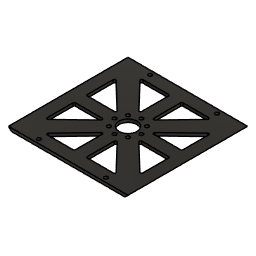
wall (Autodesk Fusion 360 design; units mm, degrees)
Autodesk Fusion 360 part; units mm, degrees
sketch "Sketch1" plane through (0, 0, 0) normal (0, 0, 1) x (1, 0, 0)
  line L0 (40, -40) -> (-60, -40)
  line L1 (-60, -40) -> (-60, 60)
  line L2 (-60, 60) -> (40, 60)
  line L3 (40, 60) -> (40, -40)
  dimension "d1" = 100
  dimension "d2" = 100
  constraint horizontal L0
  constraint vertical L1
  constraint horizontal L2
  constraint vertical L3
  measures "d1" distance of L0.start L0.end
  measures "d2" distance of L0.start L2.end
extrude "Extrude1" add sketch "Sketch1" along normal blind 2.5
sketch "Sketch2" plane through (0, 0, 2.5) normal (0, 0, 1) x (-1, 0, 0)
  line L0 (-40, -60) -> (60, -60)
  line L1 (60, -60) -> (60, 40)
  line L2 (60, 40) -> (-40, 40)
  line L3 (-40, 40) -> (-40, -60)
  point P0 (44.5, -10)
  point P1 (38, 36.5)
  point P2 (10, 36.5)
  point P3 (-18, 36.5)
  point P4 (-24.5, -10)
  point P5 (38, -56.5)
  point P6 (10, -56.5)
  point P7 (-18, -56.5)
  dimension "d7" = 50
  dimension "d11" = 50
  dimension "d12" = 28
  dimension "d13" = 28
  dimension "d14" = 3.5
  dimension "d15" = 3.5
  dimension "d16" = 3.5
  dimension "d17" = 50
  dimension "d25" = 50
  dimension "d26" = 28
  dimension "d27" = 28
  dimension "d28" = 3.5
  dimension "d29" = 3.5
  dimension "d30" = 3.5
  dimension "d34" = 15.5
  dimension "d35" = 15.5
  measures "d7" distance of L0 P0
  measures "d11" distance of L1 P2
  measures "d12" distance of P1 P2
  measures "d13" distance of P2 P3
  measures "d14" distance of L2 P1
  measures "d15" distance of L2 P2
  measures "d16" distance of L2 P3
  measures "d17" distance of L2 P4
  measures "d25" distance of L1 P6
  measures "d26" horizontal distance of P5 P6
  measures "d27" horizontal distance of P6 P7
  measures "d28" distance of L0 P6
  measures "d29" distance of L0 P5
  measures "d30" distance of L0 P7
  measures "d34" distance of L1 P0
  measures "d35" distance of L3 P4
hole "Hole1" at (-38, 56.5, 2.5) at (18, 56.5, 2.5) at (18, -36.5, 2.5) at (-38, -36.5, 2.5) direction (0, 0, -1) diameter 3 depth 10 tip angle 118
sketch "Sketch3" plane through (0, 0, 2.5) normal (0, 0, 1) x (-1, 0, 0)
  circle A0 centre (-18, 36.5) radius 1.5
  circle A1 centre (38, -56.5) radius 1.5
  circle A2 centre (-18, -56.5) radius 1.5
  circle A3 centre (38, 36.5) radius 1.5
  line L0 (-40, -60) -> (60, -60)
  line L1 (60, -60) -> (60, 40)
  line L2 (60, 40) -> (-40, 40)
  line L3 (-40, 40) -> (-40, -60)
  circle A4 centre (10, -10) radius 7.5
  dimension "d36" = 15
  measures "d36" diameter of A4
extrude "Extrude2" cut sketch "Sketch3" against normal blind 2.5 contours A4
sketch "Sketch4" plane through (0, 0, 0) normal (0, 0, 1) x (1, 0, 0)
  circle A0 centre (-10, 10) radius 15
  circle A1 centre (-10, 10) radius 7.5
  circle A2 centre (-10, 21.25) radius 1.5
  circle A3 centre (-2.045, 17.955) radius 1.5
  circle A4 centre (1.25, 10) radius 1.5
  circle A5 centre (-2.045, 2.045) radius 1.5
  circle A6 centre (-10, -1.25) radius 1.5
  circle A7 centre (-17.955, 2.045) radius 1.5
  circle A8 centre (-21.25, 10) radius 1.5
  circle A9 centre (-17.955, 17.955) radius 1.5
  point P0 (-10, 21.25)
  point P1 (-17.955, 17.955)
  point P2 (-21.25, 10)
  point P3 (-17.955, 2.045)
  point P4 (-10, -1.25)
  point P5 (-2.045, 2.045)
  point P6 (1.25, 10)
  point P7 (-2.045, 17.955)
  point P8 (-17.955, 17.955)
  point P9 (-21.25, 10)
  point P10 (-17.955, 2.045)
  point P11 (-10, -1.25)
  point P12 (-2.045, 2.045)
  point P13 (1.25, 10)
  point P14 (-2.045, 17.955)
  dimension "d39" = 30
  dimension "d40" = 11.25
  dimension "d42" = 360
  dimension "d46" = 3
  dimension "d47" = 3
  dimension "d48" = 3
  dimension "d49" = 3
  dimension "d50" = 3
  dimension "d51" = 3
  dimension "d52" = 3
  dimension "d53" = 3
  constraint coincident P0 A2.centre
  constraint coincident P14 P7
  constraint coincident P13 P6
  constraint coincident P12 P5
  constraint coincident P11 P4
  constraint coincident P10 P3
  constraint coincident P9 P2
  constraint coincident P8 P1
  measures "d39" diameter of A0
  measures "d40" distance of P0 A0.centre
  measures "d46" diameter of A2
  measures "d47" diameter of A3
  measures "d48" diameter of A4
  measures "d49" diameter of A5
  measures "d50" diameter of A6
  measures "d51" diameter of A7
  measures "d52" diameter of A8
  measures "d53" diameter of A9
extrude "Extrude3" cut sketch "Sketch4" along normal blind 9 contours A2 | A3 | A4 | A5 | A6 | A7 | A8 | A9
sketch "Sketch7" plane through (0, 0, 2.5) normal (0, 0, 1) x (-1, 0, 0)
  circle A0 centre (10, -21.25) radius 1.5
  circle A1 centre (10, 1.25) radius 1.5
  circle A2 centre (2.045, -2.045) radius 1.5
  circle A3 centre (17.955, -17.955) radius 1.5
  circle A4 centre (2.045, -17.955) radius 1.5
  circle A5 centre (17.955, -2.045) radius 1.5
  circle A6 centre (-1.25, -10) radius 1.5
  circle A7 centre (21.25, -10) radius 1.5
  circle A8 centre (10, -10) radius 7.5
  circle A9 centre (-18, 36.5) radius 1.5
  circle A10 centre (38, -56.5) radius 1.5
  circle A11 centre (-18, -56.5) radius 1.5
  circle A12 centre (38, 36.5) radius 1.5
  line L0 (-40, -60) -> (60, -60)
  line L1 (60, -60) -> (60, 40)
  line L2 (60, 40) -> (-40, 40)
  line L3 (-40, 40) -> (-40, -60)
  circle A13 centre (10, -10) radius 15
  dimension "d56" = 30
  constraint concentric A8 A13
  measures "d56" diameter of A13
sketch "Sketch8" plane through (0, 0, 2.5) normal (0, 0, 1) x (-1, 0, 0)
  line L0 (10, -10) -> (10, 40)
  line L1 (10, 40) -> (10, -60)
  constraint vertical L0
  constraint parallel L0 L1
sketch "Sketch9" plane through (0, 0, 2.5) normal (0, 0, 1) x (-1, 0, 0)
  line L0 (-40, -10) -> (60, -10)
  constraint horizontal L0
sketch "Sketch10" plane through (0, 0, 2.5) normal (0, 0, 1) x (-1, 0, 0)
  line L0 (-40, 40) -> (60, -60)
sketch "Sketch11" plane through (0, 0, 0) normal (0, 0, 1) x (1, 0, 0)
  line L0 (-60, -40) -> (40, 60)
sketch "Sketch13" plane through (0, 0, 2.5) normal (0, 0, 1) x (-1, 0, 0)
  line L0 (-17.6512, 30) -> (4, 30)
  line L1 (5, 29) -> (5, 6.4828)
  line L2 (3.2792, 5.7897) -> (-18.372, 28.3069)
  arc A0 (-17.6512, 30) -> (-18.372, 28.3069) centre (-17.6512, 29) ccw
  arc A1 (5, 29) -> (4, 30) centre (4, 29) ccw
  arc A2 (3.2792, 5.7897) -> (5, 6.4828) centre (4, 6.4828) ccw
  line L3 (-40, 40) -> (60, -60)
  arc A3 (-6.4828, -5) -> (-5.7897, -3.2792) centre (-6.4828, -4) ccw
  line L4 (-29, -5) -> (-6.4828, -5)
  line L5 (-5.7897, -3.2792) -> (-28.3069, 18.372)
  arc A4 (-28.3069, 18.372) -> (-30, 17.6512) centre (-29, 17.6512) ccw
  line L6 (-30, 17.6512) -> (-30, -4)
  arc A5 (-30, -4) -> (-29, -5) centre (-29, -4) ccw
  line L7 (-40, -10) -> (60, -10)
  line L8 (-29, -15) -> (-6.4828, -15)
  arc A6 (-5.7897, -16.7208) -> (-6.4828, -15) centre (-6.4828, -16) ccw
  line L9 (-5.7897, -16.7208) -> (-28.3069, -38.372)
  arc A7 (-30, -37.6512) -> (-28.3069, -38.372) centre (-29, -37.6512) ccw
  line L10 (-30, -37.6512) -> (-30, -16)
  arc A8 (-29, -15) -> (-30, -16) centre (-29, -16) ccw
  line L11 (60, 40) -> (-40, -60)
  line L12 (5, -49) -> (5, -26.4828)
  arc A9 (4, -50) -> (5, -49) centre (4, -49) ccw
  arc A10 (5, -26.4828) -> (3.2792, -25.7897) centre (4, -26.4828) ccw
  line L13 (3.2792, -25.7897) -> (-18.372, -48.3069)
  line L14 (-17.6512, -50) -> (4, -50)
  arc A11 (-18.372, -48.3069) -> (-17.6512, -50) centre (-17.6512, -49) ccw
  line L15 (10, 40) -> (10, -60)
  arc A12 (16.7208, -25.7897) -> (15, -26.4828) centre (16, -26.4828) ccw
  line L16 (15, -49) -> (15, -26.4828)
  line L17 (16.7208, -25.7897) -> (38.372, -48.3069)
  line L18 (37.6512, -50) -> (16, -50)
  arc A13 (15, -49) -> (16, -50) centre (16, -49) ccw
  arc A14 (37.6512, -50) -> (38.372, -48.3069) centre (37.6512, -49) ccw
  arc A15 (26.4828, -15) -> (25.7897, -16.7208) centre (26.4828, -16) ccw
  line L19 (25.7897, -16.7208) -> (48.3069, -38.372)
  line L20 (49, -15) -> (26.4828, -15)
  arc A16 (50, -16) -> (49, -15) centre (49, -16) ccw
  line L21 (50, -37.6512) -> (50, -16)
  arc A17 (48.3069, -38.372) -> (50, -37.6512) centre (49, -37.6512) ccw
  line L22 (25.7897, -3.2792) -> (48.3069, 18.372)
  arc A18 (50, 17.6512) -> (48.3069, 18.372) centre (49, 17.6512) ccw
  line L23 (50, 17.6512) -> (50, -4)
  arc A19 (49, -5) -> (50, -4) centre (49, -4) ccw
  line L24 (49, -5) -> (26.4828, -5)
  arc A20 (25.7897, -3.2792) -> (26.4828, -5) centre (26.4828, -4) ccw
  line L25 (37.6512, 30) -> (16, 30)
  arc A21 (38.372, 28.3069) -> (37.6512, 30) centre (37.6512, 29) ccw
  line L26 (16.7208, 5.7897) -> (38.372, 28.3069)
  arc A22 (15, 6.4828) -> (16.7208, 5.7897) centre (16, 6.4828) ccw
  line L27 (15, 29) -> (15, 6.4828)
  arc A23 (16, 30) -> (15, 29) centre (16, 29) ccw
  point P0 (-20, 30)
  point P1 (5, 30)
  point P2 (5, 4)
  dimension "d57" = 1
  constraint horizontal L0
  constraint perpendicular L0 L1
  constraint tangent L0 A0
  constraint tangent L2 A0
  constraint tangent L0 A1
  constraint tangent L1 A1
  constraint equal A0 A1
  constraint tangent L1 A2
  constraint tangent L2 A2
  constraint equal A0 A2
  constraint symmetric L0.start L3 A4.end
  constraint symmetric L2.end L3 L5.end
  constraint symmetric A0 L3 A4
  constraint symmetric L0.end L3 L6.end
  constraint symmetric L1.start L3 L4.start
  constraint symmetric A1 L3 A5
  constraint symmetric L1.end L3 A3.start
  constraint symmetric L2.start L3 A3.end
  constraint symmetric A2 L3 A3
  constraint symmetric A3.end L7 A6.start
  constraint symmetric A3.start L7 L8.end
  constraint symmetric A3 L7 A6
  constraint symmetric L4.start L7 L8.start
  constraint symmetric L5.end L7 L9.end
  constraint symmetric A4.end L7 A7.start
  constraint symmetric A4 L7 A7
  constraint symmetric L6.end L7 L10.end
  constraint symmetric A5 L7 A8
  constraint symmetric L8.start L11 L12.start
  constraint symmetric L8.end L11 L12.end
  constraint symmetric A6.start L11 A10.end
  constraint symmetric A6 L11 A10
  constraint symmetric L9.end L11 L13.end
  constraint symmetric A7.start L11 L14.start
  constraint symmetric A7 L11 A11
  constraint symmetric L10.end L11 A9.start
  constraint symmetric A8 L11 A9
  constraint symmetric L12.start L15 L16.start
  constraint symmetric L12.end L15 A12.end
  constraint symmetric A9.start L15 L18.end
  constraint symmetric A9 L15 A13
  constraint symmetric A10.end L15 A12.start
  constraint symmetric A10 L15 A12
  constraint symmetric L13.end L15 L17.end
  constraint symmetric L14.start L15 L18.start
  constraint symmetric A11 L15 A14
  constraint symmetric L3 A12.end A15.start
  constraint symmetric L3 A12.start A15.end
  constraint symmetric L3 A12 A15
  constraint symmetric L3 L16.start L20.start
  constraint symmetric L3 L17.end L19.end
  constraint symmetric L3 L18.start L21.start
  constraint symmetric L3 L18.end A16.start
  constraint symmetric L3 A13 A16
  constraint symmetric L3 A14 A17
  constraint symmetric L7 A15.end L22.start
  constraint symmetric L7 A15.start L24.end
  constraint symmetric L7 A15 A20
  constraint symmetric L7 L19.end L22.end
  constraint symmetric L7 L20.start A19.start
  constraint symmetric L7 A16.start L23.end
  constraint symmetric L7 A16 A19
  constraint symmetric L7 L21.start A18.start
  constraint symmetric L7 A17 A18
  constraint symmetric L11 A19.start L27.start
  constraint symmetric L11 L22.start L26.start
  constraint symmetric L11 L22.end A21.start
  constraint symmetric L11 A18.start L25.start
  constraint symmetric L11 A18 A21
  constraint symmetric L11 L23.end L25.end
  constraint symmetric L11 A19 A23
  constraint symmetric L11 L24.end A22.start
  constraint symmetric L11 A20 A22
  measures "d57" radius of A0
extrude "Extrude7" cut sketch "Sketch13" against normal blind 5
sketch "Sketch14" plane through (0, 60, 0) normal (0, 1, 0) x (-1, 0, 0)
  line L0 (-40, 0) -> (60, 0)
  line L1 (60, 0) -> (60, 2.5)
  line L2 (60, 2.5) -> (-40, 2.5)
  line L3 (-40, 2.5) -> (-40, 0)
  line L4 (-40, 2.5) -> (-37.5, 0)
  point P0 (-40, 2.5)
  point P1 (-40, 0)
  point P2 (-37.5, 0)
  point P3 (-40, 0)
  dimension "d60" = 2.5
  constraint coincident P0 L2.end
  constraint coincident P3 L0.start
  constraint coincident L0 P2
  constraint coincident P2 L4.end
  measures "d60" distance of P2 P3
extrude "Extrude5" cut sketch "Sketch14" against normal blind 104 contours L0 L3 L4
sketch "Sketch15" plane through (0, 60, 0) normal (0, 1, 0) x (-1, 0, 0)
  line L0 (-40, 2.5) -> (-37.5, 0)
  line L1 (-37.5, 0) -> (60, 0)
  line L2 (60, 0) -> (60, 2.5)
  line L3 (60, 2.5) -> (-40, 2.5)
  line L4 (60, 2.5) -> (57.5, 0)
  point P0 (60, 2.5)
  point P1 (60, 0)
  point P2 (57.5, 0)
  point P3 (60, 0)
  dimension "d63" = 2.5
  constraint coincident P0 L2.end
  constraint coincident P1 L1.end
  constraint coincident L1 P2
  constraint coincident P2 L4.end
  measures "d63" distance of P2 P3
extrude "Extrude6" cut sketch "Sketch15" against normal blind 105 contours L1 L2 L4
sketch "Sketch16" plane through (0, 0, 2.5) normal (0, 0, 1) x (-1, 0, 0)
sketch "Sketch17" plane through (0, 0, 2.5) normal (0, 0, 1) x (-1, 0, 0)
